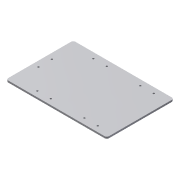
# Autodesk Inventor part: BottomSidePanel
Saved by Autodesk Inventor 2014 (Build 180170000, 170)
## iProperties
Created: 2014-08-11
Part Number: BottomSidePanel
Material: Generic
Document SubType Name: Modeling
Designer: Peele
Density: 1 g/cm^3
Appearance: White
Author: Peele
Autodesk Inventor part; units mm, degrees
ref_plane "YZ Plane" through (0, 0, 0) normal (1, 0, 0) x (0, 1, 0)
ref_plane "XZ Plane" through (0, 0, 0) normal (0, 1, 0) x (-1, 0, 0)
ref_plane "XY Plane" through (0, 0, 0) normal (0, 0, 1) x (1, 0, 0)
sketch "Sketch1" plane through (0, 0, 0) normal (0, 0, 1) x (1, 0, 0)
  line L0 (-100, -50) -> (100, -50)
  line L1 (100, -50) -> (100, 50)
  line L2 (100, 50) -> (-100, 50)
  line L3 (-100, 50) -> (-100, -50)
  line L4 (-100, -50) -> (100, 50) construction
  line L5 (100, -50) -> (-100, 50) construction
  point P0 (0, 0)
  dimension "d0" = 200
  dimension "d1" = 100
  constraints: 12 end point, 2 midpoint, 2 parallel, 1 horizontal, 1 perpendicular
  measures "d0" distance of L1.end L2.end
  measures "d1" distance of L0.end L1.end
extrude "Extrusion1" add sketch "Sketch1" along normal blind 4
sketch "Sketch2" plane through (0, 0, 4) normal (0, 0, 1) x (1, 0, 0)
  line L0 (-100, -50) -> (-125, -25)
  line L1 (-125, -25) -> (-125, 25)
  line L2 (-125, 25) -> (-100, 50)
  line L3 (-100, 50) -> (-75, 75)
  line L4 (-75, 75) -> (-30, 75)
  line L5 (-30, 75) -> (-5, 50)
  line L6 (-100, -50) -> (-75, -75)
  line L7 (-75, -75) -> (-30, -75)
  line L8 (-30, -75) -> (-5, -50)
  line L9 (-5, 50) -> (-5, -50)
  line L10 (100, 50) -> (75, 75)
  line L11 (75, 75) -> (30, 75)
  line L12 (30, 75) -> (5, 50)
  line L13 (100, 50) -> (5, 50)
  line L14 (100, -50) -> (5, -50)
  line L15 (5, -50) -> (30, -75)
  line L16 (30, -75) -> (75, -75)
  line L17 (75, -75) -> (100, -50)
  circle A0 centre (-67.5, 62.5) radius 2
  circle A1 centre (-37.5, 62.5) radius 2
  circle A2 centre (37.5, 62.5) radius 2
  circle A3 centre (67.5, 62.5) radius 2
  circle A4 centre (37.5, -62.5) radius 2
  circle A5 centre (67.5, -62.5) radius 2
  circle A6 centre (-67.5, -62.5) radius 2
  circle A7 centre (-37.5, -62.5) radius 2
  circle A8 centre (-112.5, -15) radius 2
  circle A9 centre (-112.5, 15) radius 2
  line L18 (-100, -50) -> (100, -50) projected
  point P0 (0, 0)
  dimension "d6" = 45
  dimension "d8" = 30
  dimension "d9" = 30
  dimension "d11" = 30
  dimension "d13" = 25
  dimension "d14" = 7.5
  dimension "d15" = 7.5
  dimension "d16" = 50
  dimension "d17" = 10
  dimension "d18" = 12.5
  dimension "d19" = 4
  dimension "d20" = 12.5
  dimension "d21" = 12.5
  constraints: 36 end point, 12 equal length, 10 centre point, 9 equal radius, 6 horizontal alignment, 5 vertical alignment, 4 perpendicular, 3 collinear, 2 horizontal, 2 parallel, 1 point on line
  measures "d6" distance of L3.end L4.end
  measures "d8" distance of A3.centre A2.centre
  measures "d9" distance of A0.centre A1.centre
  measures "d11" distance of A9.centre A8.centre
  measures "d13" distance between parallel lines of L11 L13
  measures "d14" horizontal distance of L11.end A2.centre
  measures "d15" horizontal distance of L4.end A1.centre
  measures "d16" distance of L0.end L1.end
  measures "d17" vertical distance of L1.end A9.centre
  measures "d18" distance from line of L1 A9.centre
  measures "d19" diameter of A3
  measures "d20" distance from line of A3.centre L13
  measures "d21" distance from line of A5.centre L14
extrude "Extrusion2" add sketch "Sketch2" against normal blind 4
sketch "Sketch3" plane through (0, 0, 4) normal (0, 0, 1) x (1, 0, 0)
  line L0 (-5, -50) -> (5, -50) projected
  line L1 (5, -50) -> (30, -75) projected
  line L2 (75, -75) -> (100, -50) projected
  line L3 (100, 50) -> (75, 75) projected
  line L4 (30, 75) -> (5, 50) projected
  line L5 (5, 50) -> (-5, 50) projected
  line L6 (-5, 50) -> (-30, 75) projected
  line L7 (-75, 75) -> (-125, 25) projected
  line L8 (-125, -25) -> (-75, -75) projected
  line L9 (-30, -75) -> (-5, -50) projected
  line L10 (-75, 75) -> (-125, 75)
  line L11 (-125, 75) -> (-125, 25)
  line L12 (-125, 25) -> (-75, 25)
  line L13 (-75, 25) -> (-75, 75)
  line L14 (-75, -75) -> (-125, -75)
  line L15 (-125, -75) -> (-125, -25)
  line L16 (-125, -25) -> (-75, -25)
  line L17 (-75, -25) -> (-75, -75)
  line L18 (-30, -75) -> (30, -75)
  line L19 (30, -75) -> (30, -50)
  line L20 (30, -50) -> (-30, -50)
  line L21 (-30, -50) -> (-30, -75)
  line L22 (-30, 75) -> (30, 75)
  line L23 (30, 75) -> (30, 50)
  line L24 (30, 50) -> (-30, 50)
  line L25 (-30, 50) -> (-30, 75)
  line L26 (75, 75) -> (100, 75)
  line L27 (100, 75) -> (100, 50)
  line L28 (100, 50) -> (75, 50)
  line L29 (75, 50) -> (75, 75)
  line L30 (100, -50) -> (75, -50)
  line L31 (75, -50) -> (75, -75)
  line L32 (75, -75) -> (100, -75)
  line L33 (100, -75) -> (100, -50)
  point P0 (0, 0)
  constraints: 48 end point, 12 parallel, 6 horizontal, 6 perpendicular, 2 collinear
extrude "Extrusion3" add sketch "Sketch3" against normal blind 4 contours L0 L1 L18 L9 | L2 L33 L32 | L3 L26 L27 | L4 L5 L6 L22 | L7 L11 L10 | L8 L14 L15
fillet "Fillet1" radius 5 4 edges at (100, 75, 2) (100, -75, 2) (-125, 75, 2) (-125, -75, 2)
equation "\"d9\" = d8"
equation "\"d14\" = -0.5 * d9 + 0.5 * d6"
equation "\"d15\" = d14"
equation "\"d17\" = -0.5 * d11 + 0.5 * d16"
body "Solid1"
